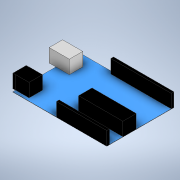
# Autodesk Inventor part: arduinoUNO
Saved by Autodesk Inventor 2020 (Build 240168000, 168)
## iProperties
Created: 2020-04-18
Part Number: arduinoUNO
Material: Genérico
Document SubType Name: Modeling
Designer: eduardoADM
Density: 1 g/cm^3
Appearance: Padrão
Author: eduardoADM
Autodesk Inventor part; units mm, degrees
note: some values were not read from the file. Chosen so that the rebuilt part matches the saved one: second side of "Extrusão4".
ref_plane "YZ Plane" through (0, 0, 0) normal (1, 0, 0) x (0, 1, 0)
ref_plane "XZ Plane" through (0, 0, 0) normal (0, 1, 0) x (-1, 0, 0)
ref_plane "XY Plane" through (0, 0, 0) normal (0, 0, 1) x (1, 0, 0)
sketch "Esboço3" plane through (0, 0, 0) normal (0, 1, 0) x (-1, 0, 0)
  line L0 (0, 0) -> (70, 0)
  line L1 (70, 0) -> (70, -50)
  line L2 (70, -50) -> (0, -50)
  line L3 (0, -50) -> (0, 0)
  dimension "d4" = 70
  dimension "d5" = 50
  constraints: 8 end point, 2 parallel, 1 horizontal, 1 perpendicular
  measures "d4" distance of L1.end L2.end
  measures "d5" distance of L0.end L1.end
extrude "Extrusão2" add sketch "Esboço3" along normal blind 0.2
sketch "Esboço4" plane through (0, 0.2, 0) normal (0, 1, 0) x (1, 0, 0)
  line L0 (0, 0) -> (0, 50) projected
  line L1 (0, 50) -> (-45, 50)
  line L2 (-45, 50) -> (-45, 48)
  line L3 (-45, 48) -> (0, 48)
  line L4 (0, 48) -> (0, 50)
  line L5 (-70, 0) -> (0, 0) projected
  line L6 (0, 0) -> (-37.5, 0)
  line L7 (-37.5, 0) -> (-37.5, 2)
  line L8 (-37.5, 2) -> (0, 2)
  line L9 (0, 2) -> (0, 0)
  line L10 (0, 2) -> (0, 12)
  line L11 (0, 12) -> (-33, 12)
  line L12 (-33, 12) -> (-33, 22)
  line L13 (-33, 22) -> (0, 22)
  line L14 (0, 22) -> (0, 12)
  dimension "d8" = 45
  dimension "d9" = 2
  dimension "d10" = 37.5
  dimension "d11" = 2
  dimension "d12" = 10
  dimension "d13" = 33
  dimension "d14" = 10
  constraints: 26 end point, 6 parallel, 3 horizontal, 3 perpendicular, 1 point on line
  measures "d8" distance of L3.end L2.end
  measures "d9" distance of L2.end L1.end
  measures "d10" distance of L7.end L8.end
  measures "d11" distance of L6.end L7.end
  measures "d12" distance of L8.end L10.end
  measures "d13" distance of L12.end L13.end
  measures "d14" distance of L11.end L12.end
extrude "Extrusão3" add sketch "Esboço4" along normal blind 10
sketch "Esboço5" plane through (0, 0.2, 0) normal (0, 1, 0) x (1, 0, 0)
  line L0 (-70, 0) -> (-70, 2.1)
  line L1 (-70, 50) -> (-70, 0) projected
  line L2 (-70, 2.1) -> (-60, 2.1)
  line L3 (-60, 2.1) -> (-60, 12.1)
  line L4 (-60, 12.1) -> (-72, 12.1)
  line L5 (-60, 2.1) -> (-72, 2.1)
  line L6 (-72, 2.1) -> (-72, 12.1)
  line L7 (-72, 12.1) -> (-60, 12.1)
  line L8 (-60, 12.1) -> (-60, 2.1)
  point P0 (0, 0)
  point P1 (-70, 12.1)
  constraints: 16 end point, 3 parallel, 2 horizontal, 2 perpendicular, 1 point on line
extrude "Extrusão4" add sketch "Esboço5" along normal blind 10 contours L4 L3 L2 L1
sketch "Esboço7" plane through (-70, 0, -50) normal (-1, 0, 0) x (0, 0, 1)
  line L0 (48, 0.2) -> (48, 10.2) projected
  line L1 (48, 0.2) -> (38, 0.2) projected
  line L2 (48, 10.2) -> (38, 10.2)
  line L3 (38, 10.2) -> (38, 0.2)
  line L4 (38, 0.2) -> (48, 0.2)
  line L5 (48, 0.2) -> (48, 10.2)
  point P0 (50, 0)
  constraints: 8 end point, 2 parallel, 1 horizontal, 1 perpendicular
extrude "Extrusão5" add sketch "Esboço7" along normal blind 2
sketch "Esboço8" plane through (0, 0.2, 0) normal (0, 1, 0) x (1, 0, 0)
  line L0 (-60, 12.1) -> (-70, 12.1) projected
  line L1 (-70, 12.1) -> (-70, 32.1)
  line L2 (-70, 50) -> (-70, 12.1) projected
  line L3 (-70, 32.1) -> (-70, 39.6)
  line L4 (-70, 32.1) -> (-60, 32.1)
  line L5 (-60, 32.1) -> (-60, 42.1)
  line L6 (-60, 42.1) -> (-70, 42.1)
  line L7 (-70, 42.1) -> (-70, 32.1)
  point P0 (0, 0)
  constraints: 12 end point, 2 parallel, 2 point on line, 1 horizontal, 1 perpendicular
extrude "Extrusão6" add sketch "Esboço8" along normal blind 10
sketch "Esboço9" plane through (-70, 0, -50) normal (-1, 0, 0) x (0, 0, 1)
  line L0 (17.9, 10.2) -> (7.9, 10.2)
  line L1 (7.9, 10.2) -> (7.9, 0.2)
  line L2 (7.9, 0.2) -> (17.9, 0.2)
  line L3 (17.9, 0.2) -> (17.9, 10.2)
  point P0 (50, 0)
  dimension "d32" = 10
  dimension "d33" = 10
  constraints: 8 end point, 2 parallel, 1 horizontal, 1 perpendicular
  measures "d32" distance of L2.end L1.end
  measures "d33" distance of L1.end L0.end
extrude "Extrusão7" add sketch "Esboço9" along normal blind 5
